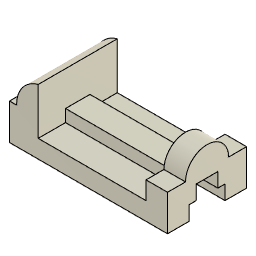
devansh2 v1 (Autodesk Fusion 360 design; units mm, degrees)
Autodesk Fusion 360 part; units mm, degrees
sketch "Sketch1" plane through (0, 0, 0) normal (0, 0, 1) x (1, 0, 0)
  line L0 (0, 0) -> (125, 0)
  line L1 (125, 0) -> (125, 65)
  line L2 (125, 65) -> (0, 65)
  line L3 (0, 65) -> (0, 0)
  constraint horizontal L0
  constraint vertical L1
  constraint horizontal L2
  constraint vertical L3
  constraint coincident L0.start L3.end
extrude "Extrude1" add sketch "Sketch1" along normal blind 30
sketch "Sketch2" plane through (0, 0, 0) normal (-1, 0, 0) x (0, -1, 0)
  line L0 (-65, 0) -> (0, 0)
  line L1 (0, 0) -> (0, 30)
  line L2 (0, 30) -> (-65, 30)
  line L3 (-65, 30) -> (-65, 0)
  line L4 (-20, 0) -> (-20, 15)
  line L5 (-20, 15) -> (-25, 15)
  line L6 (-25, 15) -> (-25, 25)
  line L7 (-25, 25) -> (-40, 25)
  line L8 (-40, 25) -> (-40, 15)
  line L9 (-40, 15) -> (-45, 15)
  line L10 (-45, 15) -> (-45, 0)
  line L11 (-45, 0) -> (-20, 0)
  dimension "d18" = 15
  dimension "d19" = 15
  constraint coincident L0 L4.start
  constraint perpendicular L0 L4
  constraint perpendicular L4 L5
  constraint perpendicular L5 L6
  constraint perpendicular L6 L7
  constraint perpendicular L5 L8
  constraint perpendicular L8 L9
  constraint coincident L0 L10.end
  constraint perpendicular L0 L10
  measures "d18" distance of L9.end L10.end
  measures "d19" distance of L4.start L4.end
extrude "Extrude2" cut sketch "Sketch2" against normal blind 125 contours L0 L4 L5 L6 L7 L8 L9 L10 L11
extrude "Extrude3" cut 1 faces at (41.6667, 0, 10) along direction (0, 1, 0) blind 5
extrude "Extrude4" cut 1 faces at (83.3333, 65, 10) along direction (0, -1, 0) blind 5
extrude "Extrude5" cut 1 faces at (0, 55, 15) along direction (1, 0, 0) blind 15
sketch "Sketch3" plane through (0, 5, 0) normal (0, -1, 0) x (1, 0, 0)
  line L0 (15, 30) -> (15, 0)
  line L1 (15, 0) -> (125, 0)
  line L2 (125, 0) -> (125, 30)
  line L3 (125, 30) -> (15, 30)
  line L4 (20, 30) -> (20, 30.5)
  arc A0 (35, 50) -> (20, 30.5) centre (40.175, 30.5) ccw
  line L5 (35, 50) -> (35, 30)
  constraint coincident L3 L4.start
  constraint perpendicular L3 L4
  constraint tangent L4 A0
  constraint coincident L3 L5.end
  constraint perpendicular L3 L5
extrude "Extrude6" add sketch "Sketch3" against normal blind 55 contours L3 L4 A0 L5
sketch "Sketch4" plane through (0, 0, 30) normal (0, 0, 1) x (-1, 0, 0)
  line L0 (-35, -60) -> (-35, -5)
  line L1 (-35, -5) -> (-125, -5)
  line L2 (-125, -5) -> (-125, -60)
  line L3 (-125, -60) -> (-35, -60)
sketch "Sketch5" plane through (125, 0, 0) normal (1, 0, 0) x (0, 1, 0)
  line L0 (60, 0) -> (60, 30)
  line L1 (60, 30) -> (5, 30)
  line L2 (5, 30) -> (5, 0)
  line L3 (5, 0) -> (20, 0)
  line L4 (20, 0) -> (20, 15)
  line L5 (20, 15) -> (25, 15)
  line L6 (25, 15) -> (25, 25)
  line L7 (25, 25) -> (40, 25)
  line L8 (40, 25) -> (40, 15)
  line L9 (40, 15) -> (45, 15)
  line L10 (45, 15) -> (45, 0)
  line L11 (45, 0) -> (60, 0)
  circle A0 centre (32.5, 30) radius 15
  dimension "d13" = 30
  constraint midpoint L1 A0.centre
  measures "d13" diameter of A0
extrude "Extrude7" add sketch "Sketch5" against normal blind 15 contours L1 A0
sketch "Sketch6" plane through (0, 0, 30) normal (0, 0, 1) x (-1, 0, 0)
  line L0 (-35, -60) -> (-110, -60)
  line L1 (-110, -60) -> (-110, -5)
  line L2 (-110, -5) -> (-35, -5)
  line L3 (-35, -5) -> (-35, -60)
  constraint horizontal L0
  constraint vertical L1
  constraint horizontal L2
  constraint vertical L3
extrude "Extrude8" cut sketch "Sketch6" against normal blind 12.5
extrude "Extrude9" cut 2 faces at (51.6667, 15, 0) (88.3333, 50, 0) along direction (0, 0, 1) blind 5
sketch "Sketch7" plane through (110, 0, 0) normal (-1, 0, 0) x (0, -1, 0)
  arc A0 (-17.5, 30) -> (-47.5, 30) centre (-32.5, 30) ccw
  line L0 (-47.5, 30) -> (-60, 30)
  line L1 (-60, 30) -> (-60, 17.5)
  line L2 (-60, 17.5) -> (-40, 17.5)
  line L3 (-40, 17.5) -> (-40, 25)
  line L4 (-40, 25) -> (-25, 25)
  line L5 (-25, 25) -> (-25, 17.5)
  line L6 (-25, 17.5) -> (-5, 17.5)
  line L7 (-5, 17.5) -> (-5, 30)
  line L8 (-5, 30) -> (-17.5, 30)
  line L9 (-40, 17.5) -> (-41, 17.5)
  line L10 (-41, 17.5) -> (-41, 26)
  line L11 (-41, 26) -> (-24, 26)
  line L12 (-24, 26) -> (-24, 17.5)
  line L13 (-24, 17.5) -> (-25, 17.5)
  line L14 (-25, 17.5) -> (-25, 25)
  line L15 (-40, 25) -> (-40, 17.5)
  dimension "d22" = 1
  dimension "d23" = 8.5
  dimension "d24" = 17
  constraint coincident L2.end L3.start
  constraint coincident L2 L9.end
  constraint perpendicular L9 L10
  constraint perpendicular L10 L11
  constraint coincident L6 L12.end
  constraint perpendicular L6 L12
  constraint coincident L5.end L6.start
  constraint coincident L4.end L5.start
  constraint coincident L3.end L4.start
  measures "d22" distance of L2.end L9.end
  measures "d23" distance of L9.end L10.end
  measures "d24" distance of L10.end L11.end
extrude "Extrude10" add sketch "Sketch7" along normal blind 75 contours L2 L3 L4 L5 L6 L9 L10 L11 L12 L13 L14 L15
